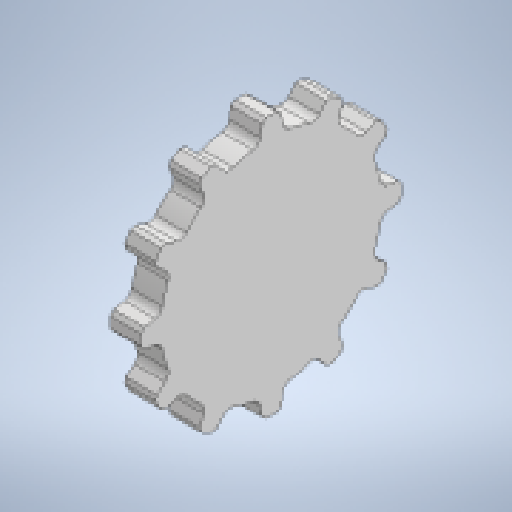
# Autodesk Inventor part: 主动轮
Saved by Autodesk Inventor 2025.1 (Build 291241000, 241)
## iProperties
Created: 2025-08-27
Part Number: 主动轮
Material: 常规
Document SubType Name: Modeling
Designer: Piw
Density: 1 g/cm^3
Appearance: 默认
Author: Piw
Autodesk Inventor part; units mm, degrees
ref_plane "YZ Plane" through (0, 0, 0) normal (1, 0, 0) x (0, 1, 0)
ref_plane "XZ Plane" through (0, 0, 0) normal (0, 1, 0) x (-1, 0, 0)
ref_plane "XY Plane" through (0, 0, 0) normal (0, 0, 1) x (1, 0, 0)
sketch "草图1" plane through (0, 0, 0) normal (1, 0, 0) x (0, 1, 0)
  circle A0 centre (0, 0) radius 25
  line L0 (29.5, 0) -> (29.5, -1.2)
  line L1 (28.7122, -2.1389) -> (26.2684, -2.5698)
  arc A1 (26.2684, -2.5698) -> (24.6441, -4.2032) centre (26.6157, -4.5394) ccw
  line L2 (31.8647, 0) -> (-37.7189, 0)
  line L3 (29.5, -1.2) -> (28.7122, -2.1389)
  line L4 (29.5, 0) -> (29.5, 1.2)
  line L5 (28.7122, 2.1389) -> (26.2684, 2.5698)
  arc A2 (24.6441, 4.2032) -> (26.2684, 2.5698) centre (26.6157, 4.5394) ccw
  line L6 (29.5, 1.2) -> (28.7122, 2.1389)
  line L7 (26.1477, 13.7108) -> (25.9349, 12.5037)
  line L8 (25.5477, 14.75) -> (26.1477, 13.7108)
  line L9 (25.9349, 12.5037) -> (24.034, 10.9086)
  line L10 (25.5477, 14.75) -> (24.9477, 15.7892)
  line L11 (24.9477, 15.7892) -> (23.796, 16.2084)
  arc A3 (24.034, 10.9086) -> (23.444, 8.682) centre (25.3196, 9.3766) ccw
  line L12 (23.796, 16.2084) -> (21.4642, 15.3597)
  arc A4 (19.2409, 15.9621) -> (21.4642, 15.3597) centre (20.7801, 17.2391) ccw
  line L13 (27.5957, 15.9324) -> (-32.6655, -18.8594)
  line L14 (15.7892, 24.9477) -> (16.2084, 23.796)
  line L15 (14.75, 25.5477) -> (15.7892, 24.9477)
  line L16 (16.2084, 23.796) -> (15.3597, 21.4642)
  line L17 (14.75, 25.5477) -> (13.7108, 26.1477)
  line L18 (13.7108, 26.1477) -> (12.5037, 25.9349)
  arc A5 (15.3597, 21.4642) -> (15.9621, 19.2409) centre (17.2391, 20.7801) ccw
  line L19 (12.5037, 25.9349) -> (10.9086, 24.034)
  arc A6 (8.682, 23.444) -> (10.9086, 24.034) centre (9.3766, 25.3196) ccw
  line L20 (15.9324, 27.5957) -> (-18.8594, -32.6655)
  line L21 (1.2, 29.5) -> (2.1389, 28.7122)
  line L22 (0, 29.5) -> (1.2, 29.5)
  line L23 (2.1389, 28.7122) -> (2.5698, 26.2684)
  line L24 (0, 29.5) -> (-1.2, 29.5)
  line L25 (-1.2, 29.5) -> (-2.1389, 28.7122)
  arc A7 (2.5698, 26.2684) -> (4.2032, 24.6441) centre (4.5394, 26.6157) ccw
  line L26 (-2.1389, 28.7122) -> (-2.5698, 26.2684)
  arc A8 (-4.2032, 24.6441) -> (-2.5698, 26.2684) centre (-4.5394, 26.6157) ccw
  line L27 (0, 31.8647) -> (0, -37.7189)
  line L28 (-13.7108, 26.1477) -> (-12.5037, 25.9349)
  line L29 (-14.75, 25.5477) -> (-13.7108, 26.1477)
  line L30 (-12.5037, 25.9349) -> (-10.9086, 24.034)
  line L31 (-14.75, 25.5477) -> (-15.7892, 24.9477)
  line L32 (-15.7892, 24.9477) -> (-16.2084, 23.796)
  arc A9 (-10.9086, 24.034) -> (-8.682, 23.444) centre (-9.3766, 25.3196) ccw
  line L33 (-16.2084, 23.796) -> (-15.3597, 21.4642)
  arc A10 (-15.9621, 19.2409) -> (-15.3597, 21.4642) centre (-17.2391, 20.7801) ccw
  line L34 (-15.9324, 27.5957) -> (18.8594, -32.6655)
  line L35 (-24.9477, 15.7892) -> (-23.796, 16.2084)
  line L36 (-25.5477, 14.75) -> (-24.9477, 15.7892)
  line L37 (-23.796, 16.2084) -> (-21.4642, 15.3597)
  line L38 (-25.5477, 14.75) -> (-26.1477, 13.7108)
  line L39 (-26.1477, 13.7108) -> (-25.9349, 12.5037)
  arc A11 (-21.4642, 15.3597) -> (-19.2409, 15.9621) centre (-20.7801, 17.2391) ccw
  line L40 (-25.9349, 12.5037) -> (-24.034, 10.9086)
  arc A12 (-23.444, 8.682) -> (-24.034, 10.9086) centre (-25.3196, 9.3766) ccw
  line L41 (-27.5957, 15.9324) -> (32.6655, -18.8594)
  line L42 (-29.5, 1.2) -> (-28.7122, 2.1389)
  line L43 (-29.5, 0) -> (-29.5, 1.2)
  line L44 (-28.7122, 2.1389) -> (-26.2684, 2.5698)
  line L45 (-29.5, 0) -> (-29.5, -1.2)
  line L46 (-29.5, -1.2) -> (-28.7122, -2.1389)
  arc A13 (-26.2684, 2.5698) -> (-24.6441, 4.2032) centre (-26.6157, 4.5394) ccw
  line L47 (-28.7122, -2.1389) -> (-26.2684, -2.5698)
  arc A14 (-24.6441, -4.2032) -> (-26.2684, -2.5698) centre (-26.6157, -4.5394) ccw
  line L48 (-31.8647, 0) -> (37.7189, 0)
  line L49 (-26.1477, -13.7108) -> (-25.9349, -12.5037)
  line L50 (-25.5477, -14.75) -> (-26.1477, -13.7108)
  line L51 (-25.9349, -12.5037) -> (-24.034, -10.9086)
  line L52 (-25.5477, -14.75) -> (-24.9477, -15.7892)
  line L53 (-24.9477, -15.7892) -> (-23.796, -16.2084)
  arc A15 (-24.034, -10.9086) -> (-23.444, -8.682) centre (-25.3196, -9.3766) ccw
  line L54 (-23.796, -16.2084) -> (-21.4642, -15.3597)
  arc A16 (-19.2409, -15.9621) -> (-21.4642, -15.3597) centre (-20.7801, -17.2391) ccw
  line L55 (-27.5957, -15.9324) -> (32.6655, 18.8594)
  line L56 (-15.7892, -24.9477) -> (-16.2084, -23.796)
  line L57 (-14.75, -25.5477) -> (-15.7892, -24.9477)
  line L58 (-16.2084, -23.796) -> (-15.3597, -21.4642)
  line L59 (-14.75, -25.5477) -> (-13.7108, -26.1477)
  line L60 (-13.7108, -26.1477) -> (-12.5037, -25.9349)
  arc A17 (-15.3597, -21.4642) -> (-15.9621, -19.2409) centre (-17.2391, -20.7801) ccw
  line L61 (-12.5037, -25.9349) -> (-10.9086, -24.034)
  arc A18 (-8.682, -23.444) -> (-10.9086, -24.034) centre (-9.3766, -25.3196) ccw
  line L62 (-15.9324, -27.5957) -> (18.8594, 32.6655)
  line L63 (-1.2, -29.5) -> (-2.1389, -28.7122)
  line L64 (0, -29.5) -> (-1.2, -29.5)
  line L65 (-2.1389, -28.7122) -> (-2.5698, -26.2684)
  line L66 (0, -29.5) -> (1.2, -29.5)
  line L67 (1.2, -29.5) -> (2.1389, -28.7122)
  arc A19 (-2.5698, -26.2684) -> (-4.2032, -24.6441) centre (-4.5394, -26.6157) ccw
  line L68 (2.1389, -28.7122) -> (2.5698, -26.2684)
  arc A20 (4.2032, -24.6441) -> (2.5698, -26.2684) centre (4.5394, -26.6157) ccw
  line L69 (0, -31.8647) -> (0, 37.7189)
  line L70 (13.7108, -26.1477) -> (12.5037, -25.9349)
  line L71 (14.75, -25.5477) -> (13.7108, -26.1477)
  line L72 (12.5037, -25.9349) -> (10.9086, -24.034)
  line L73 (14.75, -25.5477) -> (15.7892, -24.9477)
  line L74 (15.7892, -24.9477) -> (16.2084, -23.796)
  arc A21 (10.9086, -24.034) -> (8.682, -23.444) centre (9.3766, -25.3196) ccw
  line L75 (16.2084, -23.796) -> (15.3597, -21.4642)
  arc A22 (15.9621, -19.2409) -> (15.3597, -21.4642) centre (17.2391, -20.7801) ccw
  line L76 (15.9324, -27.5957) -> (-18.8594, 32.6655)
  line L77 (24.9477, -15.7892) -> (23.796, -16.2084)
  line L78 (25.5477, -14.75) -> (24.9477, -15.7892)
  line L79 (23.796, -16.2084) -> (21.4642, -15.3597)
  line L80 (25.5477, -14.75) -> (26.1477, -13.7108)
  line L81 (26.1477, -13.7108) -> (25.9349, -12.5037)
  arc A23 (21.4642, -15.3597) -> (19.2409, -15.9621) centre (20.7801, -17.2391) ccw
  line L82 (25.9349, -12.5037) -> (24.034, -10.9086)
  arc A24 (23.444, -8.682) -> (24.034, -10.9086) centre (25.3196, -9.3766) ccw
  line L83 (27.5957, -15.9324) -> (-32.6655, 18.8594)
  point P0 (29.5, -2)
  point P1 (29.5, 2)
  point P2 (26.5477, 13.0179)
  point P3 (24.5477, 16.4821)
  point P4 (16.4821, 24.5477)
  point P5 (13.0179, 26.5477)
  point P6 (2, 29.5)
  point P7 (-2, 29.5)
  point P8 (-13.0179, 26.5477)
  point P9 (-16.4821, 24.5477)
  point P10 (-24.5477, 16.4821)
  point P11 (-26.5477, 13.0179)
  point P12 (-29.5, 2)
  point P13 (-29.5, -2)
  point P14 (-26.5477, -13.0179)
  point P15 (-24.5477, -16.4821)
  point P16 (-16.4821, -24.5477)
  point P17 (-13.0179, -26.5477)
  point P18 (-2, -29.5)
  point P19 (2, -29.5)
  point P20 (13.0179, -26.5477)
  point P21 (16.4821, -24.5477)
  point P22 (24.5477, -16.4821)
  point P23 (26.5477, -13.0179)
  point P24 (23.444, 8.682)
  point P25 (15.9621, 19.2409)
  point P26 (8.682, 23.444)
  point P27 (4.2032, 24.6441)
  point P28 (-4.2032, 24.6441)
  point P29 (-8.682, 23.444)
  point P30 (-15.9621, 19.2409)
  point P31 (-19.2409, 15.9621)
  point P32 (-24.6441, 4.2032)
  point P33 (-24.6441, -4.2032)
  point P34 (-23.444, -8.682)
  point P35 (-19.2409, -15.9621)
  point P36 (-15.9621, -19.2409)
  point P37 (-8.682, -23.444)
  point P38 (-4.2032, -24.6441)
  point P39 (4.2032, -24.6441)
  point P40 (8.682, -23.444)
  point P41 (15.9621, -19.2409)
  point P42 (19.2409, -15.9621)
  point P43 (23.444, -8.682)
  dimension "d0" = 50
  dimension "d1" = 2
  dimension "d2" = 100
  dimension "d3" = 2
  dimension "d4" = 4.5
  dimension "d5" = 0.8
  dimension "d6" = 0.8
  dimension "d9" = 360
  constraints: 168 end point, 60 point on line, 48 point on circle, 24 centre point, 6 symmetric about line, 2 horizontal, 1 coincident, 1 perpendicular, 1 tangent, 1 vertical, 294 other
  measures "d1" distance of L0.start point (29.5, -2)
  measures "d2" angle of L0 L1
  measures "d3" radius of A1
  measures "d5" distance of L0.end point (29.5, -2)
  measures "d6" distance of L1.start point (29.5, -2)
extrude "拉伸1" add sketch "草图1" along normal blind 5
sketch "草图2" plane through (5, 0, 0) normal (1, 0, 0) x (0, 0, -1)
  circle A0 centre (0, 0) radius 8 construction
  circle A1 centre (-8, 0) radius 1.6
  line L0 (0, 0) -> (-16.9351, 0) construction
  circle A2 centre (0, -8) radius 1.6
  circle A3 centre (8, 0) radius 1.6
  circle A4 centre (0, 8) radius 1.6
  dimension "d13" = 16
  dimension "d14" = 3.2
  dimension "d17" = 360
  constraints: 4 centre point, 2 end point, 1 coincident, 1 horizontal, 1 horizontal alignment, 1 point on line, 11 other
  measures "d14" diameter of A1
extrude "拉伸2" cut sketch "草图2" against normal blind 5
equation "\"d6\" = d5"
